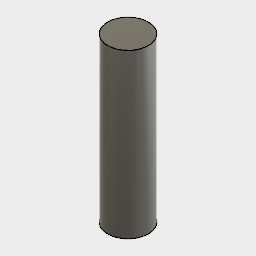
longCylinder (Autodesk Fusion 360 design; units mm, degrees)
Autodesk Fusion 360 part; units mm, degrees
sketch "Sketch2" plane through (0, 0, 0) normal (0, 1, 0) x (1, 0, 0)
  circle A0 centre (51.9635, -0.0678) radius 2.5
  dimension "d4" = 5
  measures "d4" diameter of A0
extrude "Extrude2" add sketch "Sketch2" along normal blind 20
extrude "Extrude1" [rolled back] along distance 45 taper angle 0
